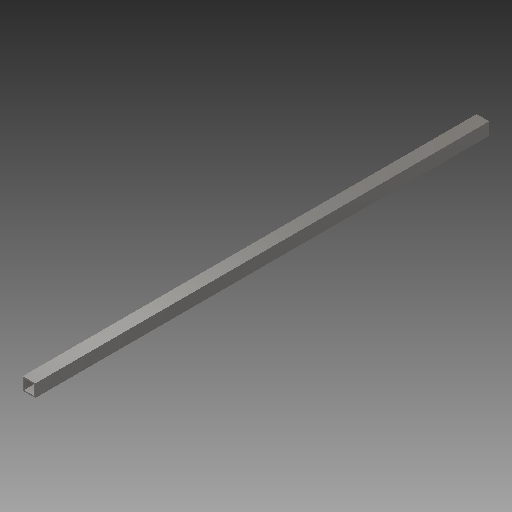
# Autodesk Inventor part: 72in2.0Sq
Saved by Autodesk Inventor 2018 (Build 220112000, 112)
## iProperties
Created: 2018-08-05
Part Number: 72in2.0Sq
Material: Steel, Mild
Document SubType Name: Modeling
Designer: Cole Tucker
Density: 7.85 g/cm^3
Appearance: Semi-Polished
Mass: 12590.5 g
Surface Area: 6753.01 cm^2
Volume: 1603.88 cm^3
Author: Cole Tucker
Autodesk Inventor part; units mm, degrees
ref_plane "YZ Plane" through (0, 0, 0) normal (1, 0, 0) x (0, 1, 0)
ref_plane "XZ Plane" through (0, 0, 0) normal (0, 1, 0) x (-1, 0, 0)
ref_plane "XY Plane" through (0, 0, 0) normal (0, 0, 1) x (1, 0, 0)
sketch "Sketch1" plane through (0, 0, 0) normal (0, 0, 1) x (1, 0, 0)
  line L0 (0, 0) -> (50.8, 0)
  line L1 (50.8, 0) -> (50.8, 50.8)
  line L2 (50.8, 50.8) -> (0, 50.8)
  line L3 (0, 50.8) -> (0, 0)
  line L4 (0, 0) -> (4.7625, 0) construction
  line L5 (4.7625, 0) -> (4.7625, 4.7625) construction
  line L6 (4.7625, 4.7625) -> (0, 4.7625) construction
  line L7 (0, 4.7625) -> (0, 0) construction
  line L8 (50.8, 50.8) -> (46.0375, 50.8) construction
  line L9 (46.0375, 50.8) -> (46.0375, 46.0375) construction
  line L10 (46.0375, 46.0375) -> (50.8, 46.0375) construction
  line L11 (50.8, 46.0375) -> (50.8, 50.8) construction
  line L12 (46.0375, 46.0375) -> (4.7625, 46.0375)
  line L13 (4.7625, 46.0375) -> (4.7625, 4.7625)
  line L14 (4.7625, 4.7625) -> (46.0375, 4.7625)
  line L15 (46.0375, 4.7625) -> (46.0375, 46.0375)
  dimension "d0" = 50.8
  dimension "d1" = 50.8
  dimension "d2" = 4.7625
  dimension "d3" = 4.7625
  dimension "d4" = 4.7625
  dimension "d5" = 4.7625
  constraints: 32 end point, 8 parallel, 4 horizontal, 4 perpendicular
  measures "d0" distance of L2.end L1.end
  measures "d1" distance of L1.end L0.end
  measures "d2" distance of L6.end L5.end
  measures "d3" distance of L5.end L4.end
  measures "d4" distance of L10.end L9.end
  measures "d5" distance of L9.end L8.end
extrude "Extrusion1" add sketch "Sketch1" along normal blind 1828.8
equation "\"d0\" = d1"
equation "\"d2\" = d3"
equation "\"d4\" = d3"
equation "\"d5\" = d3"
body "Solid1"
